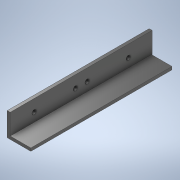
# Autodesk Inventor part: L-Bracket
Saved by Autodesk Inventor 2022 (Build 260153000, 153)
## iProperties
Created: 2021-12-05
Part Number: L-Bracket
Material: Generic
Document SubType Name: Modeling
Designer: Vedic
Density: 1 g/cm^3
Appearance: Default
Author: Vedic
Autodesk Inventor part; units mm, degrees
ref_plane "YZ Plane" through (0, 0, 0) normal (1, 0, 0) x (0, 1, 0)
ref_plane "XZ Plane" through (0, 0, 0) normal (0, 1, 0) x (-1, 0, 0)
ref_plane "XY Plane" through (0, 0, 0) normal (0, 0, 1) x (1, 0, 0)
sketch "Sketch1" plane through (0, 0, 0) normal (0, 1, 0) x (-1, 0, 0)
  line L0 (25.4, 152.4) -> (-25.4, 152.4)
  line L1 (-25.4, 152.4) -> (-25.4, -152.4)
  line L2 (-25.4, -152.4) -> (25.4, -152.4)
  line L3 (25.4, -152.4) -> (25.4, 152.4)
  point P0 (0, 0)
  dimension "d0" = 50.8
  dimension "d1" = 304.8
  dimension "d2" = 152.4
  dimension "d3" = 25.4
  constraints: 8 end point, 2 parallel, 1 horizontal, 1 perpendicular
  measures "d0" distance of L1.end L2.end
  measures "d1" distance of L2.end L0.start
  measures "d2" distance from line of L2 point (0, 0)
  measures "d3" distance from line of L3 point (0, 0)
extrude "Extrusion1" add sketch "Sketch1" along normal blind 6.35
sketch "Sketch2" plane through (0, 0, 0) normal (0, -1, 0) x (1, 0, 0)
  line L0 (-25.4, -152.4) -> (-25.4, 152.4) projected
  line L1 (-25.4, 152.4) -> (-19.05, 152.4)
  line L2 (-19.05, 152.4) -> (-19.05, -153.9502)
  line L3 (-19.05, -153.9502) -> (-25.4, -153.9502)
  line L4 (-25.4, -153.9502) -> (-25.4, 152.4)
  point P0 (0, 0)
  dimension "d6" = 6.35
  constraints: 8 end point, 2 parallel, 1 horizontal, 1 perpendicular
  measures "d6" distance of L0.end L1.end
extrude "Extrusion2" add sketch "Sketch2" against normal blind 50.8
sketch "Sketch3" plane through (-25.4, 0, -153.9502) normal (-1, 0, 0) x (0, 0, 1)
  line L0 (153.9502, 0) -> (153.1751, 50.8) construction
  line L1 (0, 50.8) -> (306.3502, 50.8) construction
  line L2 (0, 0) -> (0, 50.8) construction
  line L3 (0, 25.4) -> (306.3502, 25.4) construction
  line L4 (306.3502, 0) -> (306.3502, 50.8) construction
  circle A0 centre (165.8751, 25.4) radius 4.7625
  circle A1 centre (254.7751, 25.4) radius 4.7625
  circle A2 centre (140.4751, 25.4) radius 4.7625
  circle A3 centre (51.5751, 25.4) radius 4.7625
  point P0 (153.1751, 25.4)
  dimension "d9" = 9.525
  dimension "d10" = 12.7
  dimension "d11" = 12.7
  dimension "d12" = 101.6
  dimension "d13" = 88.9
  constraints: 4 centre point, 4 end point, 4 midpoint, 4 point on line, 3 equal radius
  measures "d9" diameter of A0
  measures "d10" distance of point (153.175, 25.4) A0.centre
  measures "d11" distance of point (153.175, 25.4) A2.centre
  measures "d12" distance of A1.centre point (153.175, 25.4)
  measures "d13" distance of A2.centre A3.centre
extrude "Extrusion3" cut sketch "Sketch3" against normal blind 50.8
equation "\"d2\" = 0.5 * d1"
equation "\"d3\" = 0.5 * d0"
equation "\"d11\" = d10"
body "Solid1"
